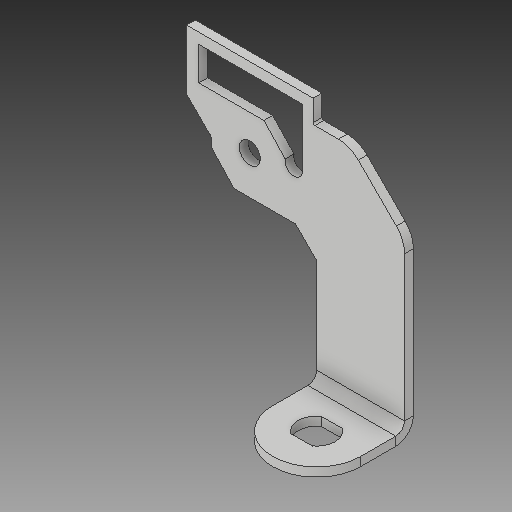
# Autodesk Inventor part: Luxcan P2
Saved by Autodesk Inventor 2018 (Build 220112000, 112)
## iProperties
Created: 2018-07-26
Part Number: Luxcan P2
Material: Generic
Document SubType Name: Sheet Metal
Designer: jocdurso
Density: 1 g/cm^3
Sheet Metal Rule: Default
Appearance: Default
Flat Pattern Width: 6.2 cm
Flat Pattern Length: 9.46549 cm
Flat Pattern Area: 58.686 cm^2
Sheet Metal Width: 62.000 mm
Sheet Metal Length: 94.655 mm
Sheet Metal Area: 5868.602 mm^2
Author: jocdurso
Autodesk Inventor part; units mm, degrees
ref_plane "YZ Plane" through (0, 0, 0) normal (1, 0, 0) x (0, 1, 0)
ref_plane "XZ Plane" through (0, 0, 0) normal (0, 1, 0) x (-1, 0, 0)
ref_plane "XY Plane" through (0, 0, 0) normal (0, 0, 1) x (1, 0, 0)
sketch "Sketch1" plane through (0, 0, 0) normal (0, 0, 1) x (1, 0, 0)
  line L0 (-12.5, 71.5) -> (12.5, 71.5)
  line L1 (12.5, 71.5) -> (12.5, 0)
  line L2 (12.5, 0) -> (-12.5, 0)
  line L3 (-12.5, 0) -> (-12.5, 71.5)
  line L4 (-49.5, 71.5) -> (12.5, 71.5)
  line L5 (12.5, 71.5) -> (12.5, 38)
  line L6 (12.5, 38) -> (-49.5, 38)
  line L7 (-49.5, 38) -> (-49.5, 71.5)
  point P0 (0, 0)
  point P1 (0, 0)
  dimension "d0" = 25
  dimension "d1" = 71.5
  dimension "d2" = 62
  dimension "d3" = 33.5
  measures "d0" distance of L0.start L0.end
  measures "d1" distance of L0.end L1.end
  measures "d2" distance of L4.start L4.end
  measures "d3" distance of L6.end L4.start
extrude "Plate1" add sketch "Sketch1" along normal blind 2.5
sketch "Sketch2" plane through (12.5, 2.5, 0) normal (0, -1, 0) x (1, 0, 0)
  line L0 (-25, 0) -> (0, 0)
  line L1 (0, 0) -> (0, 27.5)
  line L2 (0, 27.5) -> (-25, 27.5)
  line L3 (-25, 27.5) -> (-25, 0)
  constraints: 6 end point, 1 horizontal, 1 perpendicular, 1 vertical
edge flange "Flange1" height 27.5 angle 90 thickness 2.5 bend radius 2.5 thickness toward (0, -1, 0) relief tear relief width 2.5 relief depth 1.25 edges at (0, 0, 2.5) wall of the first edge with corners at (-12.5, 2.5, 0) (12.5, 2.5, 0) (12.5, 2.5, 27.5) (-12.5, 2.5, 27.5)
bend "Bend1"
corner "Corner1"
fillet "Fillet1" radius 12.5 1 edges at (-12.5, 1.25, 27.5)
fillet "Fillet2" radius 12.5 1 edges at (12.5, 1.25, 27.5)
sketch "Sketch5" plane through (-12.5, 0, 5) normal (0, -1, 0) x (1, 0, 0)
  line L0 (9.5, 14.3) -> (15.5, 14.3)
  line L1 (15.5, 14.3) -> (15.5, 5.7)
  line L2 (15.5, 5.7) -> (9.5, 5.7)
  line L3 (9.5, 5.7) -> (9.5, 14.3)
  arc A0 (25, 10) -> (0, 10) centre (12.5, 10) ccw projected
  arc A1 (9.5, 14.3) -> (9.5, 5.7) centre (12.5, 10) ccw
  arc A2 (15.5, 5.7) -> (15.5, 14.3) centre (12.5, 10) ccw
  line L4 (9.5, 5.7) -> (9.5, 14.3)
  line L5 (15.5, 5.7) -> (15.5, 14.3)
  point P0 (12.5, -5)
  point P1 (12.5, 14.3)
  point P2 (12.5, 22.5)
  dimension "d20" = 8.6
  dimension "d21" = 6
  constraints: 12 end point, 5 point on circle, 4 equal length, 2 centre point, 1 coincident, 1 horizontal, 1 midpoint, 1 perpendicular, 1 point on line, 1 vertical alignment
  measures "d20" distance of L0.end L1.end
  measures "d21" distance of L0.start L0.end
extrude "Cut1" cut sketch "Sketch5" against normal blind 2.5
sketch "Sketch6" plane through (0, 0, 2.5) normal (0, 0, 1) x (1, 0, 0)
  line L0 (12.5, 71.5) -> (-49.5, 71.5) projected
  line L1 (12.5, 71.5) -> (-13.5, 71.5)
  line L2 (-13.5, 71.5) -> (-13.5, 65)
  line L3 (-13.5, 65) -> (12.5, 65)
  line L4 (12.5, 65) -> (12.5, 71.5)
  line L5 (-3, 65) -> (12.5, 65)
  line L6 (12.5, 65) -> (12.5, 49.5)
  line L7 (12.5, 49.5) -> (-3, 65)
  point P0 (0, 0)
  dimension "d24" = 26
  dimension "d25" = 6.5
  dimension "d26" = 15.5
  dimension "d27" = 15.5
  constraints: 14 end point, 2 horizontal, 2 parallel, 2 perpendicular
  measures "d24" distance of L2.end L3.end
  measures "d25" distance of L1.end L2.end
  measures "d26" distance of L3.end L5.start
  measures "d27" distance of L3.end L6.end
extrude "Cut2" cut sketch "Sketch6" against normal blind 2.5
fillet "Fillet3" radius 0.5 1 edges at (-13.5, 65, 1.25)
fillet "Fillet4" radius 8 2 edges at (-3, 65, 1.25) (12.5, 49.5, 1.25)
sketch "Sketch7" plane through (0, 0, 2.5) normal (0, 0, 1) x (1, 0, 0)
  line L0 (-12.5, 38) -> (-49.5, 38)
  line L1 (-12.5, 38) -> (-18.5, 38)
  line L2 (-12.5, 38) -> (-12.5, 32)
  line L3 (-12.5, 5) -> (-12.5, 38)
  line L4 (-12.5, 32) -> (-18.5, 38)
  point P0 (0, 0)
  dimension "d32" = 6
  dimension "d33" = 6
  measures "d32" distance of L0.start L1.end
  measures "d33" distance of L0.start L2.end
sheet face with bend "Face2" sketch "Sketch7" thickness 2.5 toward (0, 0, -1) bend radius 2.5
bend "Bend2"
sketch "Sketch8" plane through (0, 0, 2.5) normal (0, 0, 1) x (1, 0, 0)
  line L0 (-49.5, 71.5) -> (-49.5, 38) projected
  line L1 (-49.5, 38) -> (-36, 38)
  line L2 (-18.5, 38) -> (-49.5, 38) projected
  line L3 (-49.5, 38) -> (-49.5, 54.5)
  line L4 (-49.5, 54.5) -> (-43, 54.5)
  line L5 (-49.5, 54.5) -> (-49.5, 47.5)
  line L6 (-49.5, 54.5) -> (-42.5, 47.5)
  line L7 (-36, 38) -> (-42.5, 38)
  line L8 (-36, 38) -> (-36, 45)
  line L9 (-36, 38) -> (-42.5, 45)
  line L10 (-42.5, 45) -> (-42.5, 47.5)
  point P0 (0, 0)
  dimension "d39" = 13.5
  dimension "d40" = 16.5
  dimension "d41" = 6.5
  dimension "d42" = 7
  dimension "d43" = 6.5
  dimension "d44" = 7
  constraints: 18 end point, 4 point on line, 2 vertical, 1 perpendicular
  measures "d39" distance of L0.end L1.end
  measures "d40" distance of L0.end L3.end
  measures "d41" distance of L3.end L4.end
  measures "d42" distance of L3.end L5.end
  measures "d43" distance of L1.end L7.end
  measures "d44" distance of L1.end L8.end
extrude "Cut3" cut sketch "Sketch8" against normal blind 2.5
fillet "Fillet5" radius 1 1 edges at (-42.5, 47.5, 1.25)
sketch "Sketch9" plane through (0, 0, 2.5) normal (0, 0, 1) x (1, 0, 0)
  line L0 (-49.5, 71.5) -> (-13.5, 71.5) projected
  line L1 (-49.5, 54.5) -> (-49.5, 71.5) projected
  point P0 (0, 0)
  point P1 (-31.5, 49)
  dimension "d48" = 22.5
  dimension "d49" = 18
  measures "d48" distance from line of L0 point (-31.5, 49)
  measures "d49" distance from line of point (-31.5, 49) L1
hole "Hole1" at (-31.5, 49, 2.5) direction (0, 0, -1) diameter 6 end through all
sketch "Sketch10" plane through (0, 0, 2.5) normal (0, 0, 1) x (1, 0, 0)
  line L0 (-46, 68.5) -> (-16.5, 68.5)
  line L1 (-16.5, 68.5) -> (-16.5, 59)
  line L2 (-16.5, 59) -> (-46, 59)
  line L3 (-46, 59) -> (-46, 68.5)
  line L4 (-49.5, 54.5) -> (-49.5, 71.5) projected
  line L5 (-16.5, 59) -> (-27.5, 59)
  line L6 (-16.5, 59) -> (-16.5, 52)
  circle A0 centre (-19, 52) radius 2.5
  line L7 (-49.5, 71.5) -> (-13.5, 71.5) projected
  line L8 (-21.4366, 52.5597) -> (-27.5, 59)
  point P0 (0, 0)
  dimension "d57" = 29.5
  dimension "d58" = 9.5
  dimension "d59" = 3.5
  dimension "d60" = 3
  dimension "d61" = 11
  dimension "d63" = 5
  dimension "d64" = 19.5
  dimension "d65" = 30.5
  constraints: 14 end point, 2 parallel, 2 point on circle, 1 centre point, 1 horizontal, 1 perpendicular, 1 point on line, 1 vertical
  measures "d57" distance of L0.start L0.end
  measures "d58" distance of L2.end L0.start
  measures "d59" distance between parallel lines of L4 L3
  measures "d60" distance from line of L4.end L0
  measures "d61" distance of L1.end L5.end
  measures "d63" diameter of A0
  measures "d64" distance from line of A0.centre L7
  measures "d65" distance from line of L4 A0.centre
extrude "Cut4" cut sketch "Sketch10" against normal blind 2.5
equation "\"d22\" = Thickness"
equation "\"d28\" = Thickness"
equation "\"d45\" = Thickness"
equation "\"d55\" = Thickness"
equation "\"d66\" = Thickness"
equation "\"d68\" = Thickness"
equation "\"d5\" = BendReliefWidth"
equation "\"d6\" = BendReliefDepth"
equation "\"d7\" = MinimumRemnant"
equation "\"d8\" = BendRadius"
equation "\"d11\" = BendRadius"
equation "\"d12\" = CornerReliefSize"
equation "\"d13\" = GapSize"
equation "\"d14\" = JacobiRadiusSize"
equation "\"d34\" = BendRadius"
equation "\"d35\" = BendReliefWidth"
equation "\"d37\" = MinimumRemnant"
equation "\"d36\" = BendReliefDepth"
equation "\"d38\" = BendRadius"
equation "\"BendRadius\" = Thickness"
equation "\"BendReliefWidth\" = Thickness"
equation "\"BendReliefDepth\" = 0.5 * Thickness"
equation "\"MinimumRemnant\" = 2 * Thickness"
equation "\"TransitionRadius\" = BendRadius"
equation "\"JacobiRadiusSize\" = BendRadius"
equation "\"GapSize\" = Thickness"
equation "\"d4\" = BendRadius"
equation "\"Thickness\" = 2.5"
equation "\"CornerReliefSize\" = 10"
body "Solid1"
